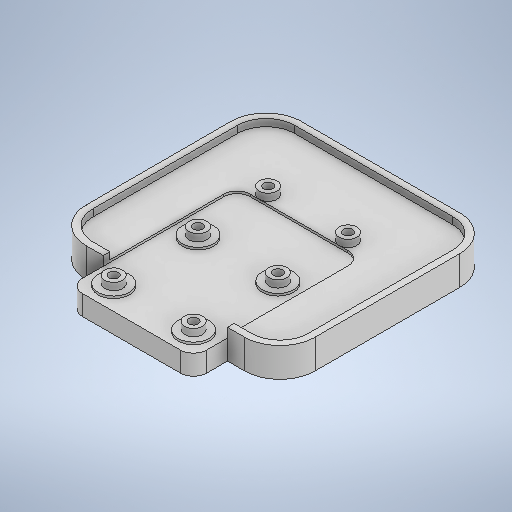
# Autodesk Inventor part: Pin-Base
Saved by Autodesk Inventor 2025 (Build 290162000, 162)
## iProperties
Created: 2025-03-04
Part Number: Pin-Base
Material: Generic
Document SubType Name: Modeling
Designer: maxsm
Density: 1 g/cm^3
Appearance: Default
Author: maxsm
Autodesk Inventor part; units mm, degrees
ref_plane "YZ Plane" through (0, 0, 0) normal (1, 0, 0) x (0, 1, 0)
ref_plane "XZ Plane" through (0, 0, 0) normal (0, 1, 0) x (-1, 0, 0)
ref_plane "XY Plane" through (0, 0, 0) normal (0, 0, 1) x (1, 0, 0)
sketch "Sketch1" plane through (0, 0, 0) normal (0, 1, 0) x (-1, 0, 0)
  line L0 (17.8, 24.25) -> (-17.8, 24.25)
  line L1 (-25.8, 16.25) -> (-25.8, -16.25)
  line L2 (-17.8, -24.25) -> (17.8, -24.25)
  line L3 (25.8, -16.25) -> (25.8, 16.25)
  line L4 (25.8, 24.25) -> (-25.8, -24.25) construction
  line L5 (-25.8, 24.25) -> (25.8, -24.25) construction
  line L6 (14, 24.25) -> (-14, 24.25)
  line L7 (-14, 24.25) -> (-14, 28.9)
  line L8 (-11, 31.9) -> (11, 31.9)
  line L9 (14, 28.9) -> (14, 24.25)
  line L10 (0, -37.5925) -> (0, 44.207) projected
  arc A0 (14, 28.9) -> (11, 31.9) centre (11, 28.9) ccw
  arc A1 (-11, 31.9) -> (-14, 28.9) centre (-11, 28.9) ccw
  arc A2 (17.8, -24.25) -> (25.8, -16.25) centre (17.8, -16.25) ccw
  arc A3 (-25.8, -16.25) -> (-17.8, -24.25) centre (-17.8, -16.25) ccw
  arc A4 (-17.8, 24.25) -> (-25.8, 16.25) centre (-17.8, 16.25) ccw
  arc A5 (25.8, 16.25) -> (17.8, 24.25) centre (17.8, 16.25) ccw
  point P0 (0, 0)
  point P1 (-14, 31.9)
  dimension "d0" = 48.5
  dimension "d1" = 51.6
  dimension "d2" = 7.65
  dimension "d3" = 28
  dimension "d5" = 3
  dimension "d10" = 8
  constraints: 20 end point, 12 point on circle, 12 tangent, 11 point on line, 6 centre point, 4 equal radius, 4 parallel, 2 horizontal, 2 midpoint, 2 perpendicular, 1 other
  measures "d0" distance of L4.end L5.start
  measures "d1" distance between parallel lines of L1 L3
  measures "d2" distance of L6.end point (-14, 31.9)
  measures "d3" distance between parallel lines of L7 L9
  measures "d5" radius of A0
  measures "d10" radius of A2
extrude "Extrusion1" add sketch "Sketch1" along normal blind 5
shell "Shell1" thickness 1.5 removed faces 1 at (-4.6667, 0, -8.0833)
sketch "Sketch2" plane through (0, 5, 0) normal (0, 1, 0) x (1, 0, 0)
  circle A0 centre (-9, -7.9) radius 1.05
  circle A1 centre (9, -7.9) radius 1.05
  circle A2 centre (-9, 7.9) radius 1.05
  circle A3 centre (9, 7.9) radius 1.05
  line L0 (-36.12, 0) -> (36.12, 0) projected
  line L1 (0, 35.48) -> (0, -43.13) projected
  circle A4 centre (-9, -26.9) radius 1.05
  circle A5 centre (9, -26.9) radius 1.05
  point P0 (0, 0)
  dimension "d11" = 2.1
  dimension "d12" = 18
  dimension "d13" = 15.8
  dimension "d14" = 19
  constraints: 6 centre point, 5 equal radius, 4 vertical alignment, 3 horizontal alignment, 2 symmetric about line
  measures "d11" diameter of A0
  measures "d12" distance of A1.centre A0.centre
  measures "d13" distance of A3.centre A1.centre
  measures "d14" distance of A0.centre A4.centre
extrude "Extrusion2" cut sketch "Sketch2" against normal through all
sketch "Sketch3" plane through (0, 5, 0) normal (0, 1, 0) x (1, 0, 0)
  circle A0 centre (9, -7.9) radius 1.05 projected
  circle A1 centre (-9, 7.9) radius 1.05 projected
  circle A2 centre (9, -26.9) radius 1.05 projected
  circle A3 centre (-9, -7.9) radius 1.05 projected
  circle A4 centre (9, 7.9) radius 1.05 projected
  circle A5 centre (-9, -26.9) radius 1.05 projected
  arc A6 (11, -31.9) -> (14, -28.9) centre (11, -28.9) ccw projected
  line L0 (11, -31.9) -> (-11, -31.9) projected
  arc A7 (-14, -28.9) -> (-11, -31.9) centre (-11, -28.9) ccw projected
  line L1 (-14, -28.9) -> (-14, -24.25) projected
  line L2 (-14, -24.25) -> (-17.8, -24.25) projected
  arc A8 (-25.8, -16.25) -> (-17.8, -24.25) centre (-17.8, -16.25) ccw projected
  line L3 (-25.8, -16.25) -> (-25.8, 16.25) projected
  arc A9 (-17.8, 24.25) -> (-25.8, 16.25) centre (-17.8, 16.25) ccw projected
  line L4 (-17.8, 24.25) -> (17.8, 24.25) projected
  arc A10 (25.8, 16.25) -> (17.8, 24.25) centre (17.8, 16.25) ccw projected
  line L5 (25.8, 16.25) -> (25.8, -16.25) projected
  arc A11 (17.8, -24.25) -> (25.8, -16.25) centre (17.8, -16.25) ccw projected
  line L6 (17.8, -24.25) -> (14, -24.25) projected
  line L7 (14, -24.25) -> (14, -28.9) projected
  line L8 (-24.3, 16.25) -> (-24.3, -16.25)
  arc A12 (-24.3, -16.25) -> (-17.8, -22.75) centre (-17.8, -16.25) ccw
  line L9 (-17.8, -22.75) -> (-12.5, -22.75)
  line L10 (-12.5, -22.75) -> (-12.5, -28.9)
  arc A13 (-12.5, -28.9) -> (-11, -30.4) centre (-11, -28.9) ccw
  line L11 (-11, -30.4) -> (11, -30.4)
  arc A14 (11, -30.4) -> (12.5, -28.9) centre (11, -28.9) ccw
  line L12 (12.5, -28.9) -> (12.5, -22.75)
  line L13 (12.5, -22.75) -> (17.8, -22.75)
  arc A15 (17.8, -22.75) -> (24.3, -16.25) centre (17.8, -16.25) ccw
  line L14 (24.3, -16.25) -> (24.3, 16.25)
  arc A16 (24.3, 16.25) -> (17.8, 22.75) centre (17.8, 16.25) ccw
  line L15 (17.8, 22.75) -> (-17.8, 22.75)
  arc A17 (-17.8, 22.75) -> (-24.3, 16.25) centre (-17.8, 16.25) ccw
  line L16 (-14, -24.25) -> (-14, -22.75)
  line L17 (14, -24.25) -> (14, -22.75)
  point P0 (0, 0)
  dimension "d17" = 1.5
  constraints: 20 end point, 12 point on circle, 6 centre point, 3 point on line, 1 perpendicular, 13 other
  measures "d17" distance between parallel lines of L3 L8
extrude "Extrusion3" add sketch "Sketch3" along normal blind 1.6 contours L17 L13 A15 L14 A16 L15 A17 L8 A12 L9 L16 L2 A8 L3 A9 L4 A10 L5 A11 L6
sketch "Sketch4" plane through (0, 5, 0) normal (0, 1, 0) x (1, 0, 0)
  circle A0 centre (-9, 7.9) radius 2
  circle A1 centre (9, 7.9) radius 2
  circle A2 centre (9, -7.9) radius 2
  circle A3 centre (-9, -7.9) radius 2
  circle A4 centre (-9, -26.9) radius 2
  circle A5 centre (9, -26.9) radius 2
  circle A6 centre (9, 7.9) radius 1.05 projected
  circle A7 centre (9, -7.9) radius 1.05 projected
  circle A8 centre (9, -26.9) radius 1.05 projected
  circle A9 centre (-9, -26.9) radius 1.05 projected
  circle A10 centre (-9, -7.9) radius 1.05 projected
  circle A11 centre (-9, 7.9) radius 1.05 projected
  point P0 (0, 0)
  dimension "d20" = 4
  constraints: 6 centre point, 6 concentric, 5 equal radius
  measures "d20" diameter of A0
extrude "Extrusion4" add sketch "Sketch4" along normal blind 1.6
sketch "Sketch5" plane through (0, 5, 0) normal (0, 1, 0) x (1, 0, 0)
  line L0 (-11, 5.9) -> (11, 5.9)
  line L1 (14, 2.9) -> (14, -28.9)
  line L2 (11, -31.9) -> (-11, -31.9)
  line L3 (-14, -28.9) -> (-14, 2.9)
  line L4 (-11, -31.9) -> (11, -31.9) projected
  line L5 (0, 35.48) -> (0, -43.13) projected
  circle A0 centre (-9, 7.9) radius 1.05 projected
  arc A1 (-11, 5.9) -> (-14, 2.9) centre (-11, 2.9) ccw
  arc A2 (14, 2.9) -> (11, 5.9) centre (11, 2.9) ccw
  arc A3 (11, -31.9) -> (14, -28.9) centre (11, -28.9) ccw
  arc A4 (-14, -28.9) -> (-11, -31.9) centre (-11, -28.9) ccw
  arc A5 (-14, -28.9) -> (-11, -31.9) centre (-11, -28.9) ccw projected
  circle A6 centre (9, -7.9) radius 2 projected
  circle A7 centre (-9, 7.9) radius 2 projected
  circle A8 centre (9, -26.9) radius 2 projected
  circle A9 centre (-9, -7.9) radius 2 projected
  circle A10 centre (9, 7.9) radius 2 projected
  circle A11 centre (-9, -26.9) radius 2 projected
  circle A12 centre (9, -7.9) radius 1.05 projected
  circle A13 centre (-9, 7.9) radius 1.05 projected
  circle A14 centre (9, -26.9) radius 1.05 projected
  circle A15 centre (-9, -7.9) radius 1.05 projected
  circle A16 centre (9, 7.9) radius 1.05 projected
  circle A17 centre (-9, -26.9) radius 1.05 projected
  arc A18 (11, -31.9) -> (14, -28.9) centre (11, -28.9) ccw projected
  line L6 (11, -31.9) -> (-11, -31.9) projected
  arc A19 (-14, -28.9) -> (-11, -31.9) centre (-11, -28.9) ccw projected
  line L7 (-14, -28.9) -> (-14, -24.25) projected
  line L8 (-14, -22.75) -> (-14, -24.25) projected
  line L9 (-17.8, -22.75) -> (-14, -22.75) projected
  arc A20 (-24.3, -16.25) -> (-17.8, -22.75) centre (-17.8, -16.25) ccw projected
  line L10 (-24.3, 16.25) -> (-24.3, -16.25) projected
  arc A21 (-17.8, 22.75) -> (-24.3, 16.25) centre (-17.8, 16.25) ccw projected
  line L11 (17.8, 22.75) -> (-17.8, 22.75) projected
  arc A22 (24.3, 16.25) -> (17.8, 22.75) centre (17.8, 16.25) ccw projected
  line L12 (24.3, -16.25) -> (24.3, 16.25) projected
  arc A23 (17.8, -22.75) -> (24.3, -16.25) centre (17.8, -16.25) ccw projected
  line L13 (14, -22.75) -> (17.8, -22.75) projected
  line L14 (14, -24.25) -> (14, -22.75) projected
  line L15 (17.8, -24.25) -> (14, -24.25) projected
  arc A24 (17.8, -24.25) -> (25.8, -16.25) centre (17.8, -16.25) ccw projected
  line L16 (25.8, 16.25) -> (25.8, -16.25) projected
  arc A25 (25.8, 16.25) -> (17.8, 24.25) centre (17.8, 16.25) ccw projected
  line L17 (-17.8, 24.25) -> (17.8, 24.25) projected
  arc A26 (-17.8, 24.25) -> (-25.8, 16.25) centre (-17.8, 16.25) ccw projected
  line L18 (-25.8, -16.25) -> (-25.8, 16.25) projected
  arc A27 (-25.8, -16.25) -> (-17.8, -24.25) centre (-17.8, -16.25) ccw projected
  line L19 (-14, -24.25) -> (-17.8, -24.25) projected
  line L20 (14, -24.25) -> (14, -28.9) projected
  circle A28 centre (-9, -26.9) radius 3.5
  circle A29 centre (-9, -7.9) radius 3.5
  circle A30 centre (9, -7.9) radius 3.5
  circle A31 centre (9, -26.9) radius 3.5
  circle A32 centre (-9, 7.9) radius 2 projected
  point P0 (0, 0)
  point P1 (0, -31.9)
  dimension "d25" = 7
  constraints: 10 tangent, 8 centre point, 8 end point, 8 point on circle, 6 equal radius, 4 coincident, 2 midpoint, 2 parallel, 2 point on line, 1 horizontal, 1 perpendicular
  measures "d25" diameter of A28
extrude "Extrusion5" cut sketch "Sketch5" against normal blind 0.5 contours L0 L5 L2 A4 L3 A1 | L0 A2 L1 A3 L2 L5
body "Solid1"
